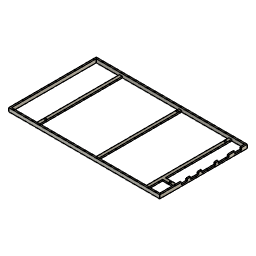
Mini PC Case V2 (Autodesk Fusion 360 design; units mm, degrees)
Autodesk Fusion 360 part; units mm, degrees
sketch "Sketch1" plane through (0, 0, 0) normal (0, 0, 1) x (1, 0, 0)
  line L0 (0, 0) -> (210, 0)
  line L1 (210, 0) -> (210, 120)
  line L2 (210, 120) -> (0, 120)
  line L3 (0, 120) -> (0, 0)
  line L4 (190, 120) -> (190, 0) construction
  line L5 (119, 120) -> (119, 0) construction
  line L6 (119, 113) -> (210, 113) construction
  line L7 (119, 24) -> (210, 24) construction
  line L8 (119, 116) -> (210, 116) construction
  circle A0 centre (119, 116) radius 1.5
  circle A1 centre (190, 113) radius 1.5
  line L9 (-2, 122) -> (-2, -2)
  line L10 (-2, -2) -> (212, -2)
  line L11 (212, -2) -> (212, 122)
  line L12 (212, 122) -> (-2, 122)
  line L13 (117, 120) -> (117, 0)
  line L14 (121, 120) -> (121, 0)
  line L15 (188, 120) -> (188, 0)
  line L16 (192, 120) -> (192, 0)
  line L17 (35, 120) -> (35, 0) construction
  line L18 (33, 120) -> (33, 0)
  line L19 (37, 120) -> (37, 0)
  line L20 (201, 120) -> (201, 0) construction
  circle A2 centre (201, 24) radius 1.5
  line L21 (118.5, 22) -> (210, 22)
  line L22 (118.5, 26) -> (210, 26)
  line L23 (35, 120) -> (35, 0) construction
  circle A3 centre (35, 13) radius 1.5
  line L24 (210, 113.8) -> (212, 113.8)
  line L25 (210, 104.5) -> (212, 104.5)
  line L26 (210, 96) -> (212, 96)
  line L27 (210, 81) -> (212, 81)
  line L28 (210, 77) -> (212, 77)
  line L29 (210, 58) -> (212, 58)
  line L30 (210, 53) -> (212, 53)
  line L31 (210, 42) -> (212, 42)
  line L32 (210, 37) -> (212, 37)
  line L33 (210, 29) -> (212, 29)
  dimension "d1" = 210
  dimension "d2" = 120
  dimension "d3" = 20
  dimension "d4" = 91
  dimension "d5" = 7
  dimension "d6" = 96
  dimension "d7" = 4
  dimension "d8" = 3
  dimension "d9" = 3
  dimension "d11" = 2
  dimension "d12" = 2
  dimension "d13" = -2
  dimension "d14" = 2
  dimension "d15" = -2
  dimension "d17" = 2
  dimension "d18" = -2
  dimension "d21" = 9
  dimension "d24" = 3
  dimension "d25" = 2
  dimension "d26" = -2
  dimension "d29" = 3
  dimension "d31" = 107
  dimension "d32" = 175
  dimension "d33" = 6.2
  dimension "d34" = 15.5
  dimension "d35" = 24
  dimension "d36" = 39
  dimension "d37" = 43
  dimension "d38" = 62
  dimension "d39" = 67
  dimension "d40" = 78
  dimension "d41" = 83
  dimension "d42" = 91
  constraint horizontal L0
  constraint vertical L1
  constraint horizontal L2
  constraint vertical L3
  constraint coincident L0.start L3.end
  constraint coincident L2 L4.start
  constraint coincident L0 L4.end
  constraint perpendicular L0 L4
  constraint coincident L2 L5.start
  constraint coincident L0 L5.end
  constraint perpendicular L0 L5
  constraint coincident L5 L6.start
  constraint coincident L1 L6.end
  constraint perpendicular L1 L6
  constraint coincident L5 L7.start
  constraint coincident L1 L7.end
  constraint perpendicular L1 L7
  constraint coincident L5 L8.start
  constraint coincident L1 L8.end
  constraint perpendicular L1 L8
  constraint coincident L8.start A0.centre
  constraint coincident L4 A1.centre
  constraint coincident L6 A1.centre
  constraint coincident L2 L17.start
  constraint coincident L0 L17.end
  constraint perpendicular L0 L17
  constraint coincident L2 L20.start
  constraint coincident L0 L20.end
  constraint perpendicular L0 L20
  constraint coincident L20 A2.centre
  constraint coincident L7 A2.centre
  constraint perpendicular L0 L23
  constraint coincident L23 A3.centre
  constraint coincident L1 L24.start
  constraint coincident L11 L24.end
  constraint perpendicular L11 L24
  constraint coincident L1 L25.start
  constraint coincident L11 L25.end
  constraint perpendicular L11 L25
  constraint coincident L1 L26.start
  constraint coincident L11 L26.end
  constraint perpendicular L11 L26
  constraint coincident L1 L27.start
  constraint coincident L11 L27.end
  constraint perpendicular L11 L27
  constraint coincident L1 L28.start
  constraint coincident L11 L28.end
  constraint perpendicular L11 L28
  constraint coincident L1 L29.start
  constraint coincident L11 L29.end
  constraint perpendicular L11 L29
  constraint coincident L1 L30.start
  constraint coincident L11 L30.end
  constraint perpendicular L11 L30
  constraint coincident L1 L31.start
  constraint coincident L11 L31.end
  constraint perpendicular L11 L31
  constraint coincident L1 L32.start
  constraint coincident L11 L32.end
  constraint perpendicular L11 L32
  constraint coincident L1 L33.start
  constraint coincident L11 L33.end
  constraint perpendicular L11 L33
  measures "d1" distance of L0.start L0.end
  measures "d2" distance of L0.start L2.end
  measures "d3" distance of L1 L4
  measures "d4" distance of L1 L5
  measures "d5" distance of L2 L6
  measures "d6" distance of L2 L7
  measures "d7" distance of L2 L8
  measures "d8" diameter of A0
  measures "d9" diameter of A1
  measures "d21" distance of L1 L20
  measures "d24" diameter of A2
  measures "d29" diameter of A3
  measures "d31" distance of L2 A3.centre
  measures "d32" distance of L1 L17
  measures "d33" distance of L1.end L24
  measures "d34" distance of L1.end L25
  measures "d35" distance of L1.end L26
  measures "d36" distance of L1.end L27
  measures "d37" distance of L1.end L28
  measures "d38" distance of L1.end L29
  measures "d39" distance of L1.end L30
  measures "d40" distance of L1.end L31
  measures "d41" distance of L1.end L32
  measures "d42" distance of L1.end L33
extrude "Extrude1" add sketch "Sketch1" along normal blind 2 contours L0 L1 L2 L3 L9 L10 L11 L12 L24 L33 | L0 L2 L18 L19 | L0 L2 L13 L14 | L0 L15 L16 L21 | L15 L16 L21 L22 | L2 L15 L16 L22 | L1 L16 L21 L22 | L1 L11 L24 L25 | L1 L11 L32 L33 | L1 L11 L25 L26 | L1 L11 L31 L32 | L1 L11 L26 L27 | L1 L11 L30 L31 | L1 L11 L27 L28 | L1 L11 L29 L30 | L1 L11 L28 L29
extrude "Extrude2" add sketch "Sketch1" along normal blind 5 contours L0 L1 L2 L3 L9 L10 L11 L12 L24 L33 | L1 L11 L25 L26 | L1 L11 L31 L32 | L1 L11 L27 L28 | L1 L11 L29 L30
